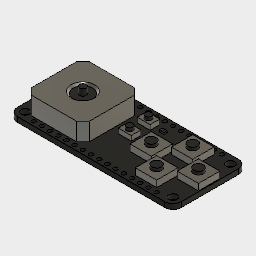
3632 Joy FeatherWing (Autodesk Fusion 360 design; units mm, degrees)
Autodesk Fusion 360 part; units mm, degrees
sketch "PCB" plane through (0, 0, 0) normal (0, 0, 1) x (1, 0, 0)
  arc A0 (50.8, 20.32) -> (48.26, 22.86) centre (48.26, 20.32) ccw
  arc A1 (48.26, 0) -> (50.8, 2.54) centre (48.26, 2.54) ccw
  line L0 (2.54, 22.86) -> (48.26, 22.86)
  line L1 (0, 20.32) -> (0, 2.54)
  circle A2 centre (5.43, 5.43) radius 0.8
  arc A3 (0, 2.54) -> (2.54, 0) centre (2.54, 2.54) ccw
  line L2 (48.26, 0) -> (2.54, 0)
  arc A4 (0, 2.54) -> (2.54, 0) centre (2.54, 2.54) ccw
  circle A5 centre (17.43, 17.43) radius 0.8
  arc A6 (50.8, 20.32) -> (48.26, 22.86) centre (48.26, 20.32) ccw
  line L3 (50.8, 2.54) -> (50.8, 20.32)
  arc A7 (48.26, 0) -> (50.8, 2.54) centre (48.26, 2.54) ccw
  line L4 (50.8, 20.32) -> (50.8, 2.54)
  line L5 (2.54, 0) -> (48.26, 0)
  arc A8 (2.54, 22.86) -> (0, 20.32) centre (2.54, 20.32) ccw
  arc A9 (2.54, 22.86) -> (0, 20.32) centre (2.54, 20.32) ccw
  line L6 (48.26, 22.86) -> (2.54, 22.86)
  line L7 (0, 2.54) -> (0, 20.32)
  circle A10 centre (2.54, 2.54) radius 1.27
  circle A11 centre (2.54, 20.32) radius 1.27
  circle A12 centre (2.43, 13.43) radius 0.635
  circle A13 centre (2.43, 11.43) radius 0.635
  circle A14 centre (2.43, 9.43) radius 0.635
  circle A15 centre (9.43, 20.43) radius 0.635
  circle A16 centre (11.43, 20.43) radius 0.635
  circle A17 centre (13.43, 20.43) radius 0.635
  circle A18 centre (48.26, 20.32) radius 1.27
  circle A19 centre (48.26, 2.54) radius 1.27
  circle A20 centre (6.35, 1.27) radius 0.635
  circle A21 centre (8.89, 1.27) radius 0.635
  circle A22 centre (11.43, 1.27) radius 0.635
  circle A23 centre (13.97, 1.27) radius 0.635
  circle A24 centre (16.51, 1.27) radius 0.635
  circle A25 centre (19.05, 1.27) radius 0.635
  circle A26 centre (21.59, 1.27) radius 0.635
  circle A27 centre (24.13, 1.27) radius 0.635
  circle A28 centre (26.67, 1.27) radius 0.635
  circle A29 centre (29.21, 1.27) radius 0.635
  circle A30 centre (31.75, 1.27) radius 0.635
  circle A31 centre (34.29, 1.27) radius 0.635
  circle A32 centre (36.83, 1.27) radius 0.635
  circle A33 centre (39.37, 1.27) radius 0.635
  circle A34 centre (41.91, 1.27) radius 0.635
  circle A35 centre (44.45, 1.27) radius 0.635
  circle A36 centre (16.51, 21.59) radius 0.635
  circle A37 centre (19.05, 21.59) radius 0.635
  circle A38 centre (21.59, 21.59) radius 0.635
  circle A39 centre (24.13, 21.59) radius 0.635
  circle A40 centre (26.67, 21.59) radius 0.635
  circle A41 centre (29.21, 21.59) radius 0.635
  circle A42 centre (31.75, 21.59) radius 0.635
  circle A43 centre (34.29, 21.59) radius 0.635
  circle A44 centre (36.83, 21.59) radius 0.635
  circle A45 centre (39.37, 21.59) radius 0.635
  circle A46 centre (41.91, 21.59) radius 0.635
  circle A47 centre (44.45, 21.59) radius 0.635
  dimension "d1" = 2.54
  dimension "d2" = 2.54
  dimension "d3" = 1.27
  dimension "d4" = 1.27
  dimension "d5" = 1.27
  dimension "d6" = 1.27
  dimension "d7" = 1.27
  dimension "d8" = 1.27
  dimension "d9" = 2.54
  dimension "d10" = 2.54
  dimension "d11" = 1.27
  dimension "d14" = 2.54
  dimension "d15" = 0
  dimension "d16" = 1.27
  dimension "d19" = 2.54
  dimension "d20" = 0
  measures "d1" diameter of A10
  measures "d2" diameter of A11
  measures "d3" diameter of A12
  measures "d4" diameter of A13
  measures "d5" diameter of A14
  measures "d6" diameter of A15
  measures "d7" diameter of A16
  measures "d8" diameter of A17
  measures "d9" diameter of A18
  measures "d10" diameter of A19
  measures "d11" diameter of A20
  measures "d16" diameter of A36
extrude "Extrude1" add sketch "PCB" along normal blind 1.6 makes body 1
sketch "thumbstick" plane through (0, 0, 1.6) normal (0, 0, 1) x (-1, 0, 0)
  circle A0 centre (-31.75, -21.59) radius 0.635
  circle A1 centre (-8.89, -1.27) radius 0.635
  circle A2 centre (-19.05, -1.27) radius 0.635
  circle A3 centre (-16.51, -1.27) radius 0.635
  circle A4 centre (-41.91, -21.59) radius 0.635
  circle A5 centre (-2.54, -2.54) radius 1.27 construction
  circle A6 centre (-39.37, -21.59) radius 0.635
  circle A7 centre (-24.13, -1.27) radius 0.635
  circle A8 centre (-13.97, -1.27) radius 0.635
  circle A9 centre (-36.83, -21.59) radius 0.635
  circle A10 centre (-48.26, -2.54) radius 1.27
  circle A11 centre (-6.35, -1.27) radius 0.635
  circle A12 centre (-11.43, -1.27) radius 0.635
  circle A13 centre (-2.43, -13.43) radius 0.635 construction
  circle A14 centre (-2.54, -20.32) radius 1.27 construction
  circle A15 centre (-44.45, -21.59) radius 0.635
  circle A16 centre (-17.43, -17.43) radius 0.8 construction
  circle A17 centre (-11.43, -20.43) radius 0.635 construction
  circle A18 centre (-9.43, -20.43) radius 0.635 construction
  circle A19 centre (-34.29, -1.27) radius 0.635
  circle A20 centre (-24.13, -21.59) radius 0.635
  circle A21 centre (-2.43, -9.43) radius 0.635 construction
  circle A22 centre (-31.75, -1.27) radius 0.635
  circle A23 centre (-2.43, -11.43) radius 0.635 construction
  circle A24 centre (-21.59, -1.27) radius 0.635
  circle A25 centre (-16.51, -21.59) radius 0.635
  circle A26 centre (-48.26, -20.32) radius 1.27
  circle A27 centre (-21.59, -21.59) radius 0.635
  circle A28 centre (-39.37, -1.27) radius 0.635
  circle A29 centre (-29.21, -1.27) radius 0.635
  circle A30 centre (-41.91, -1.27) radius 0.635
  circle A31 centre (-13.43, -20.43) radius 0.635 construction
  circle A32 centre (-34.29, -21.59) radius 0.635
  circle A33 centre (-26.67, -1.27) radius 0.635
  circle A34 centre (-26.67, -21.59) radius 0.635
  circle A35 centre (-19.05, -21.59) radius 0.635
  circle A36 centre (-44.45, -1.27) radius 0.635
  circle A37 centre (-36.83, -1.27) radius 0.635
  circle A38 centre (-29.21, -21.59) radius 0.635
  circle A39 centre (-5.43, -5.43) radius 0.8 construction
  line L0 (-2.54, 0) -> (-48.26, 0)
  arc A40 (-48.26, 0) -> (-50.8, -2.54) centre (-48.26, -2.54) ccw
  line L1 (-50.8, -2.54) -> (-50.8, -20.32)
  arc A41 (-50.8, -20.32) -> (-48.26, -22.86) centre (-48.26, -20.32) ccw
  line L2 (-48.26, -22.86) -> (-2.54, -22.86)
  arc A42 (-2.54, -22.86) -> (0, -20.32) centre (-2.54, -20.32) ccw
  line L3 (0, -20.32) -> (0, -2.54)
  arc A43 (0, -2.54) -> (-2.54, 0) centre (-2.54, -2.54) ccw
  line L4 (-20.43, -2.43) -> (-2.43, -2.43)
  line L5 (-2.43, -2.43) -> (-2.43, -20.43)
  line L6 (-2.43, -20.43) -> (-20.43, -20.43)
  line L7 (-20.43, -20.43) -> (-20.43, -2.43)
  line L8 (-20.43, -2.43) -> (-2.43, -20.43) construction
  line L9 (-2.43, -2.43) -> (-20.43, -20.43) construction
  point P0 (-11.43, -11.43)
  dimension "d23" = 18
  dimension "d24" = 18
  dimension "d25" = 11.43
  dimension "d26" = 11.43
  measures "d23" distance of L5.end L6.end
  measures "d24" distance of L4.end L5.end
  measures "d25" distance of L3 P0
  measures "d26" distance of L0 P0
extrude "Extrude2" add sketch "thumbstick" along normal blind 5.5 separate body contours L4 L5 L6 L7 makes body 2
chamfer "Chamfer1" distance 2 angle 45 4 edges at (2.43, 2.43, 4.35) (2.43, 20.43, 4.35) (20.43, 20.43, 4.35) (20.43, 2.43, 4.35) on bodies 2
sketch "stem" plane through (0, 0, 7.1) normal (0, 0, 1) x (-1, 0, 0)
  line L0 (-18.43, -2.43) -> (-20.43, -4.43)
  line L1 (-20.43, -4.43) -> (-20.43, -18.43)
  line L2 (-20.43, -18.43) -> (-18.43, -20.43)
  line L3 (-18.43, -20.43) -> (-4.43, -20.43)
  line L4 (-4.43, -20.43) -> (-2.43, -18.43)
  line L5 (-2.43, -18.43) -> (-2.43, -4.43)
  line L6 (-2.43, -4.43) -> (-4.43, -2.43)
  line L7 (-4.43, -2.43) -> (-18.43, -2.43)
  line L8 (-11.43, -20.43) -> (-11.43, -2.43) construction
  line L9 (-2.43, -11.43) -> (-20.43, -11.43) construction
  circle A0 centre (-11.43, -11.43) radius 3
  circle A1 centre (-11.43, -11.43) radius 1
  dimension "d30" = 6
  dimension "d34" = 2
  measures "d30" diameter of A0
  measures "d34" diameter of A1
extrude "Extrude3" cut sketch "stem" against normal blind 0.6 contours A0 | A1 bodies 2
chamfer "Chamfer2" distance 0.6 angle 45 1 edges at (14.227, 10.3452, 7.1) on bodies 2
extrude "Extrude4" add sketch "stem" along normal blind 2 from surface at -0.6 contours A1 bodies 2
sketch "select reset" plane through (0, 0, 1.6) normal (0, 0, 1) x (-1, 0, 0)
  circle A0 centre (-31.75, -21.59) radius 0.635
  circle A1 centre (-8.89, -1.27) radius 0.635
  circle A2 centre (-19.05, -1.27) radius 0.635
  circle A3 centre (-16.51, -1.27) radius 0.635
  circle A4 centre (-41.91, -21.59) radius 0.635
  circle A5 centre (-2.54, -2.54) radius 1.27
  circle A6 centre (-39.37, -21.59) radius 0.635
  circle A7 centre (-24.13, -1.27) radius 0.635
  circle A8 centre (-13.97, -1.27) radius 0.635
  circle A9 centre (-36.83, -21.59) radius 0.635
  circle A10 centre (-48.26, -2.54) radius 1.27
  circle A11 centre (-6.35, -1.27) radius 0.635
  circle A12 centre (-11.43, -1.27) radius 0.635
  circle A13 centre (-2.43, -13.43) radius 0.635
  circle A14 centre (-2.54, -20.32) radius 1.27
  circle A15 centre (-44.45, -21.59) radius 0.635
  circle A16 centre (-17.43, -17.43) radius 0.8
  circle A17 centre (-11.43, -20.43) radius 0.635
  circle A18 centre (-9.43, -20.43) radius 0.635
  circle A19 centre (-34.29, -1.27) radius 0.635
  circle A20 centre (-24.13, -21.59) radius 0.635
  circle A21 centre (-2.43, -9.43) radius 0.635
  circle A22 centre (-31.75, -1.27) radius 0.635
  circle A23 centre (-2.43, -11.43) radius 0.635
  circle A24 centre (-21.59, -1.27) radius 0.635
  circle A25 centre (-16.51, -21.59) radius 0.635
  circle A26 centre (-48.26, -20.32) radius 1.27
  circle A27 centre (-21.59, -21.59) radius 0.635
  circle A28 centre (-39.37, -1.27) radius 0.635
  circle A29 centre (-29.21, -1.27) radius 0.635
  circle A30 centre (-41.91, -1.27) radius 0.635
  circle A31 centre (-13.43, -20.43) radius 0.635
  circle A32 centre (-34.29, -21.59) radius 0.635
  circle A33 centre (-26.67, -1.27) radius 0.635
  circle A34 centre (-26.67, -21.59) radius 0.635
  circle A35 centre (-19.05, -21.59) radius 0.635
  circle A36 centre (-44.45, -1.27) radius 0.635
  circle A37 centre (-36.83, -1.27) radius 0.635
  circle A38 centre (-29.21, -21.59) radius 0.635
  circle A39 centre (-5.43, -5.43) radius 0.8
  line L0 (-2.54, 0) -> (-48.26, 0)
  arc A40 (-48.26, 0) -> (-50.8, -2.54) centre (-48.26, -2.54) ccw
  line L1 (-50.8, -2.54) -> (-50.8, -20.32)
  arc A41 (-50.8, -20.32) -> (-48.26, -22.86) centre (-48.26, -20.32) ccw
  line L2 (-48.26, -22.86) -> (-2.54, -22.86)
  arc A42 (-2.54, -22.86) -> (0, -20.32) centre (-2.54, -20.32) ccw
  line L3 (0, -20.32) -> (0, -2.54)
  arc A43 (0, -2.54) -> (-2.54, 0) centre (-2.54, -2.54) ccw
  line L4 (-26.765, -16.915) -> (-22.765, -16.915)
  line L5 (-22.765, -16.915) -> (-22.765, -19.915)
  line L6 (-22.765, -19.915) -> (-26.765, -19.915)
  line L7 (-26.765, -19.915) -> (-26.765, -16.915)
  line L8 (-26.765, -16.915) -> (-22.765, -19.915) construction
  line L9 (-22.765, -16.915) -> (-26.765, -19.915) construction
  line L10 (-26.765, -11.073) -> (-22.765, -11.073)
  line L11 (-22.765, -11.073) -> (-22.765, -14.073)
  line L12 (-22.765, -14.073) -> (-26.765, -14.073)
  line L13 (-26.765, -14.073) -> (-26.765, -11.073)
  line L14 (-26.765, -11.073) -> (-22.765, -14.073) construction
  line L15 (-22.765, -11.073) -> (-26.765, -14.073) construction
  circle A44 centre (-24.765, -18.415) radius 1
  circle A45 centre (-24.765, -12.573) radius 1
  point P0 (-24.765, -18.415)
  point P1 (-24.765, -12.573)
  dimension "d38" = 4
  dimension "d39" = 3
  dimension "d40" = 24.765
  dimension "d41" = 18.415
  dimension "d42" = 4
  dimension "d43" = 3
  dimension "d44" = 24.765
  dimension "d45" = 12.573
  dimension "d48" = 2
  dimension "d49" = 2
  measures "d38" distance of L5.end L6.end
  measures "d39" distance of L4.end L5.end
  measures "d40" distance of L3 P0
  measures "d41" distance of L0 P0
  measures "d42" distance of L11.end L12.end
  measures "d43" distance of L10.end L11.end
  measures "d44" distance of L3 P1
  measures "d45" distance of L0 P1
  measures "d48" diameter of A44
  measures "d49" diameter of A45
extrude "Extrude5" add sketch "select reset" along normal blind 1.5 separate body contours L4 L5 L6 L7 | L10 L11 L12 L13 | A44 | A45 makes body 3 at (25.4317, 17.915, 1.6) makes body 4 at (25.4317, 12.073, 1.6)
extrude "Extrude6" add sketch "select reset" along normal blind 1 from surface at 1.5 contours A44 | A45 bodies 3 4
sketch "action buttons" plane through (0, 0, 1.6) normal (0, 0, 1) x (-1, 0, 0)
  circle A0 centre (-31.75, -21.59) radius 0.635
  circle A1 centre (-8.89, -1.27) radius 0.635
  circle A2 centre (-19.05, -1.27) radius 0.635
  circle A3 centre (-16.51, -1.27) radius 0.635
  circle A4 centre (-41.91, -21.59) radius 0.635
  circle A5 centre (-2.54, -2.54) radius 1.27
  circle A6 centre (-39.37, -21.59) radius 0.635
  circle A7 centre (-24.13, -1.27) radius 0.635
  circle A8 centre (-13.97, -1.27) radius 0.635
  circle A9 centre (-36.83, -21.59) radius 0.635
  circle A10 centre (-48.26, -2.54) radius 1.27
  circle A11 centre (-6.35, -1.27) radius 0.635
  circle A12 centre (-11.43, -1.27) radius 0.635
  circle A13 centre (-2.43, -13.43) radius 0.635
  circle A14 centre (-2.54, -20.32) radius 1.27
  circle A15 centre (-44.45, -21.59) radius 0.635
  circle A16 centre (-17.43, -17.43) radius 0.8
  circle A17 centre (-11.43, -20.43) radius 0.635
  circle A18 centre (-9.43, -20.43) radius 0.635
  circle A19 centre (-34.29, -1.27) radius 0.635
  circle A20 centre (-24.13, -21.59) radius 0.635
  circle A21 centre (-2.43, -9.43) radius 0.635
  circle A22 centre (-31.75, -1.27) radius 0.635
  circle A23 centre (-2.43, -11.43) radius 0.635
  circle A24 centre (-21.59, -1.27) radius 0.635
  circle A25 centre (-16.51, -21.59) radius 0.635
  circle A26 centre (-48.26, -20.32) radius 1.27
  circle A27 centre (-21.59, -21.59) radius 0.635
  circle A28 centre (-39.37, -1.27) radius 0.635
  circle A29 centre (-29.21, -1.27) radius 0.635
  circle A30 centre (-41.91, -1.27) radius 0.635
  circle A31 centre (-13.43, -20.43) radius 0.635
  circle A32 centre (-34.29, -21.59) radius 0.635
  circle A33 centre (-26.67, -1.27) radius 0.635
  circle A34 centre (-26.67, -21.59) radius 0.635
  circle A35 centre (-19.05, -21.59) radius 0.635
  circle A36 centre (-44.45, -1.27) radius 0.635
  circle A37 centre (-36.83, -1.27) radius 0.635
  circle A38 centre (-29.21, -21.59) radius 0.635
  circle A39 centre (-5.43, -5.43) radius 0.8
  line L0 (-2.54, 0) -> (-48.26, 0)
  arc A40 (-48.26, 0) -> (-50.8, -2.54) centre (-48.26, -2.54) ccw
  line L1 (-50.8, -2.54) -> (-50.8, -20.32)
  arc A41 (-50.8, -20.32) -> (-48.26, -22.86) centre (-48.26, -20.32) ccw
  line L2 (-48.26, -22.86) -> (-2.54, -22.86)
  arc A42 (-2.54, -22.86) -> (0, -20.32) centre (-2.54, -20.32) ccw
  line L3 (0, -20.32) -> (0, -2.54)
  arc A43 (0, -2.54) -> (-2.54, 0) centre (-2.54, -2.54) ccw
  line L4 (-35.939, -8.13) -> (-29.339, -8.13)
  line L5 (-29.339, -8.13) -> (-29.339, -14.73)
  line L6 (-29.339, -14.73) -> (-35.939, -14.73)
  line L7 (-35.939, -14.73) -> (-35.939, -8.13)
  line L8 (-35.939, -8.13) -> (-29.339, -14.73) construction
  line L9 (-29.339, -8.13) -> (-35.939, -14.73) construction
  line L10 (-43.178, -13.718) -> (-36.578, -13.718)
  line L11 (-36.578, -13.718) -> (-36.578, -20.318)
  line L12 (-36.578, -20.318) -> (-43.178, -20.318)
  line L13 (-43.178, -20.318) -> (-43.178, -13.718)
  line L14 (-43.178, -13.718) -> (-36.578, -20.318) construction
  line L15 (-36.578, -13.718) -> (-43.178, -20.318) construction
  line L16 (-43.178, -2.542) -> (-36.578, -2.542)
  line L17 (-36.578, -2.542) -> (-36.578, -9.142)
  line L18 (-36.578, -9.142) -> (-43.178, -9.142)
  line L19 (-43.178, -9.142) -> (-43.178, -2.542)
  line L20 (-43.178, -2.542) -> (-36.578, -9.142) construction
  line L21 (-36.578, -2.542) -> (-43.178, -9.142) construction
  line L22 (-50.544, -8.13) -> (-43.944, -8.13)
  line L23 (-43.944, -8.13) -> (-43.944, -14.73)
  line L24 (-43.944, -14.73) -> (-50.544, -14.73)
  line L25 (-50.544, -14.73) -> (-50.544, -8.13)
  line L26 (-50.544, -8.13) -> (-43.944, -14.73) construction
  line L27 (-43.944, -8.13) -> (-50.544, -14.73) construction
  circle A44 centre (-32.639, -11.43) radius 1.5
  circle A45 centre (-39.878, -17.018) radius 1.5
  circle A46 centre (-39.878, -5.842) radius 1.5
  circle A47 centre (-47.244, -11.43) radius 1.5
  point P0 (-32.639, -11.43)
  point P1 (-39.878, -17.018)
  point P2 (-39.878, -5.842)
  point P3 (-47.244, -11.43)
  dimension "d53" = 6.6
  dimension "d54" = 6.6
  dimension "d55" = 32.639
  dimension "d56" = 11.43
  dimension "d57" = 6.6
  dimension "d58" = 6.6
  dimension "d59" = 39.878
  dimension "d60" = 17.018
  dimension "d61" = 6.6
  dimension "d62" = 6.6
  dimension "d63" = 39.878
  dimension "d64" = 5.842
  dimension "d65" = 6.6
  dimension "d66" = 6.6
  dimension "d67" = 11.43
  dimension "d68" = 47.244
  dimension "d69" = 3
  dimension "d70" = 3
  dimension "d71" = 3
  dimension "d72" = 3
  measures "d53" distance of L5.end L6.end
  measures "d54" distance of L4.end L5.end
  measures "d55" distance of L3 P0
  measures "d56" distance of L0 P0
  measures "d57" distance of L11.end L12.end
  measures "d58" distance of L10.end L11.end
  measures "d59" distance of L3 P1
  measures "d60" distance of L0 P1
  measures "d61" distance of L17.end L18.end
  measures "d62" distance of L16.end L17.end
  measures "d63" distance of L3 P2
  measures "d64" distance of L0 P2
  measures "d65" distance of L22.end L23.end
  measures "d66" distance of L23.end L24.end
  measures "d67" distance of L0 P3
  measures "d68" distance of L3 P3
  measures "d69" diameter of A44
  measures "d70" diameter of A45
  measures "d71" diameter of A46
  measures "d72" diameter of A47
extrude "Extrude7" add sketch "action buttons" along normal blind 2 separate body contours L4 L5 L6 L7 | L10 L11 L12 L13 | L16 L17 L18 L19 | L22 L23 L24 L25 | A44 | A45 | A46 | A47 makes body 5 at (33.739, 10.33, 1.6) makes body 6 at (40.978, 6.942, 1.6) makes body 7 at (40.978, 18.118, 1.6) makes body 8 at (48.344, 10.33, 1.6)
extrude "Extrude8" add sketch "action buttons" along normal blind 1 from surface at 2 contours A44 | A45 | A46 | A47 bodies 5 6 7 8
sketch "Act LED" plane through (0, 0, 1.6) normal (0, 0, 1) x (-1, 0, 0)
  circle A0 centre (-31.75, -21.59) radius 0.635
  circle A1 centre (-8.89, -1.27) radius 0.635
  circle A2 centre (-19.05, -1.27) radius 0.635
  circle A3 centre (-16.51, -1.27) radius 0.635
  circle A4 centre (-41.91, -21.59) radius 0.635
  circle A5 centre (-2.54, -2.54) radius 1.27
  circle A6 centre (-39.37, -21.59) radius 0.635
  circle A7 centre (-24.13, -1.27) radius 0.635
  circle A8 centre (-13.97, -1.27) radius 0.635
  circle A9 centre (-36.83, -21.59) radius 0.635
  circle A10 centre (-48.26, -2.54) radius 1.27
  circle A11 centre (-6.35, -1.27) radius 0.635
  circle A12 centre (-11.43, -1.27) radius 0.635
  circle A13 centre (-2.43, -13.43) radius 0.635
  circle A14 centre (-2.54, -20.32) radius 1.27
  circle A15 centre (-44.45, -21.59) radius 0.635
  circle A16 centre (-17.43, -17.43) radius 0.8
  circle A17 centre (-11.43, -20.43) radius 0.635
  circle A18 centre (-9.43, -20.43) radius 0.635
  circle A19 centre (-34.29, -1.27) radius 0.635
  circle A20 centre (-24.13, -21.59) radius 0.635
  circle A21 centre (-2.43, -9.43) radius 0.635
  circle A22 centre (-31.75, -1.27) radius 0.635
  circle A23 centre (-2.43, -11.43) radius 0.635
  circle A24 centre (-21.59, -1.27) radius 0.635
  circle A25 centre (-16.51, -21.59) radius 0.635
  circle A26 centre (-48.26, -20.32) radius 1.27
  circle A27 centre (-21.59, -21.59) radius 0.635
  circle A28 centre (-39.37, -1.27) radius 0.635
  circle A29 centre (-29.21, -1.27) radius 0.635
  circle A30 centre (-41.91, -1.27) radius 0.635
  circle A31 centre (-13.43, -20.43) radius 0.635
  circle A32 centre (-34.29, -21.59) radius 0.635
  circle A33 centre (-26.67, -1.27) radius 0.635
  circle A34 centre (-26.67, -21.59) radius 0.635
  circle A35 centre (-19.05, -21.59) radius 0.635
  circle A36 centre (-44.45, -1.27) radius 0.635
  circle A37 centre (-36.83, -1.27) radius 0.635
  circle A38 centre (-29.21, -21.59) radius 0.635
  circle A39 centre (-5.43, -5.43) radius 0.8
  line L0 (-2.54, 0) -> (-48.26, 0)
  arc A40 (-48.26, 0) -> (-50.8, -2.54) centre (-48.26, -2.54) ccw
  line L1 (-50.8, -2.54) -> (-50.8, -20.32)
  arc A41 (-50.8, -20.32) -> (-48.26, -22.86) centre (-48.26, -20.32) ccw
  line L2 (-48.26, -22.86) -> (-2.54, -22.86)
  arc A42 (-2.54, -22.86) -> (0, -20.32) centre (-2.54, -20.32) ccw
  line L3 (0, -20.32) -> (0, -2.54)
  arc A43 (0, -2.54) -> (-2.54, 0) centre (-2.54, -2.54) ccw
  line L4 (-30.087, -17.915) -> (-28.587, -17.915)
  line L5 (-28.587, -17.915) -> (-28.587, -18.915)
  line L6 (-28.587, -18.915) -> (-30.087, -18.915)
  line L7 (-30.087, -18.915) -> (-30.087, -17.915)
  line L8 (-30.087, -17.915) -> (-28.587, -18.915) construction
  line L9 (-28.587, -17.915) -> (-30.087, -18.915) construction
  point P0 (-29.337, -18.415)
  dimension "d78" = 1
  dimension "d79" = 1.5
  dimension "d80" = 29.337
  dimension "d81" = 18.415
  measures "d78" distance of L4.end L5.end
  measures "d79" distance of L5.end L6.end
  measures "d80" distance of L3 P0
  measures "d81" distance of L0 P0
extrude "Extrude9" add sketch "Act LED" along normal blind 0.5 separate body contours L4 L5 L6 L7 makes body 9
named bodies: "pcb", "thumbstick", "select", "reset", "LED"
